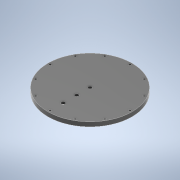
# Autodesk Inventor part: Platform
Saved by Autodesk Inventor 2022 (Build 260153000, 153)
## iProperties
Created: 2022-02-20
Part Number: Platform
Material: Genérico
Document SubType Name: Modeling
Designer: JK
Density: 1 g/cm^3
Appearance: Suave - Negro
Author: JK
Autodesk Inventor part; units mm, degrees
ref_plane "YZ Plane" through (0, 0, 0) normal (1, 0, 0) x (0, 1, 0)
ref_plane "XZ Plane" through (0, 0, 0) normal (0, 1, 0) x (-1, 0, 0)
ref_plane "XY Plane" through (0, 0, 0) normal (0, 0, 1) x (1, 0, 0)
sketch "Boceto1" plane through (0, 0, 0) normal (0, 1, 0) x (-1, 0, 0)
  circle A0 centre (0, 0) radius 62.862
  circle A1 centre (0, 0) radius 52.5
  dimension "d0" = 125.724
  dimension "d1" = 105
  constraints: 2 centre point, 2 coincident
  measures "d0" diameter of A0
  measures "d1" diameter of A1
extrude "Extrusión1" add sketch "Boceto1" along normal blind 23
sketch "Boceto2" plane through (0, 23, 0) normal (0, 1, 0) x (1, 0, 0)
  circle A0 centre (0, 0) radius 52.5 projected
extrude "Extrusión2" add sketch "Boceto2" against normal blind 5
sketch "Boceto3" plane through (0, 23, 0) normal (0, 1, 0) x (1, 0, 0)
  circle A0 centre (0, 0) radius 2.65
  dimension "d6" = 5.3
  constraints: 1 centre point, 1 coincident
  measures "d6" diameter of A0
extrude "Extrusión3" cut sketch "Boceto3" against normal through all
sketch "Boceto4" plane through (0, 23, 0) normal (0, 1, 0) x (1, 0, 0)
  circle A0 centre (-59.612, 0) radius 1.65
  point P0 (0, 0)
  dimension "d9" = 3.3
  dimension "d10" = 59.612
  constraints: 1 centre point
  measures "d9" diameter of A0
  measures "d10" distance of A0.centre point (0, 0)
extrude "Extrusión4" cut sketch "Boceto4" against normal through all
pattern_circular "Patrón circular1" count 12 over 360 about axis through (0, 0, 0) along (0, 1, 0) of "Extrusión4"
fillet "Empalme1" radius 3 1 edges at (52.5, 18, 0)
sketch "Boceto6" plane through (0, 23, 0) normal (0, 1, 0) x (1, 0, 0)
  circle A0 centre (0, -59.612) radius 1.65 projected
  circle A1 centre (0, -59.612) radius 2.85
  line L0 (1.6454, -62.462) -> (-1.6454, -62.462)
  line L1 (-1.6454, -62.462) -> (-3.2909, -59.612)
  line L2 (-3.2909, -59.612) -> (-1.6454, -56.762)
  line L3 (-1.6454, -56.762) -> (1.6454, -56.762)
  line L4 (1.6454, -56.762) -> (3.2909, -59.612)
  line L5 (3.2909, -59.612) -> (1.6454, -62.462)
  point P0 (0, 0)
  dimension "d20" = 5.7
  constraints: 12 end point, 2 coincident, 1 centre point, 1 horizontal alignment, 1 tangent, 13 other
  measures "d20" diameter of A1
extrude "Extrusión6" [suppressed]
pattern_circular "Patrón circular2" [suppressed]
sketch "Boceto10" plane through (0, 0, 0) normal (0, -1, 0) x (1, 0, 0)
  circle A0 centre (0, 0) radius 2.65 projected
  circle A1 centre (0, 0) radius 81.3362
  constraints: 1 centre point, 1 coincident
extrude "Extrusión10" cut sketch "Boceto10" against normal blind 16.5
sketch "Boceto11" plane through (0, 23, 0) normal (0, 1, 0) x (1, 0, 0)
  circle A0 centre (0, -20) radius 2.7
  circle A1 centre (0, -40) radius 2.7
  point P0 (0, 0)
  dimension "d40" = 5.4
  dimension "d41" = 20
  dimension "d42" = 20
  constraints: 2 centre point, 1 equal radius
  measures "d40" diameter of A0
  measures "d41" distance of A0.centre A1.centre
  measures "d42" distance of point (0, 0) A0.centre
extrude "Extrusión11" cut sketch "Boceto11" against normal through all
sketch "Boceto12" plane through (0, 18, 0) normal (0, -1, 0) x (1, 0, 0)
  circle A0 centre (0, 0) radius 2.65 projected
  circle A1 centre (0, 0) radius 5
  circle A2 centre (0, 20) radius 2.7 projected
  circle A3 centre (0, 20) radius 5
  circle A4 centre (0, 40) radius 2.7 projected
  circle A5 centre (0, 40) radius 5
  dimension "d45" = 10
  constraints: 3 centre point, 3 coincident, 2 equal radius
  measures "d45" diameter of A1
extrude "Extrusión12" cut sketch "Boceto12" against normal blind 2 contours A0 | A1 | A2 | A3 | A4 | A5
sketch "Boceto9" plane through (0, 18, 0) normal (0, -1, 0) x (1, 0, 0)
  circle A0 centre (0, 0) radius 2.65 projected
  circle A1 centre (0, 0) radius 74.2803
  constraints: 1 centre point, 1 coincident
sketch "Boceto8" plane through (0, 0, 0) normal (0, -1, 0) x (1, 0, 0)
  circle A0 centre (0, 0) radius 2.65 projected
  circle A1 centre (0, 0) radius 69.5586
  constraints: 1 centre point, 1 coincident
sketch "Boceto7" plane through (0, 0, 0) normal (0, -1, 0) x (1, 0, 0)
  line L0 (0, 0) -> (-67.2382, 47.1765)
  line L1 (-67.2382, 47.1765) -> (-46.5407, 66.6024)
  circle A0 centre (0, 0) radius 2.65 projected
  line L2 (-46.5407, 66.6024) -> (0, 0)
  line L3 (0, 0) -> (-86.5562, 0)
  line L4 (0, 0) -> (-56.8894, 56.8894)
  point P0 (-1.5179, 2.1722)
  point P1 (-2.1693, 1.5221)
  dimension "d26" = 20
  dimension "d28" = 45
  constraints: 10 end point, 1 horizontal, 1 midpoint
  measures "d26" angle of L2 L0
  measures "d28" angle of L3 L4
